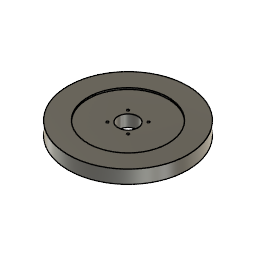
part - rotation base (Autodesk Fusion 360 design; units mm, degrees)
Autodesk Fusion 360 part; units mm, degrees
sketch "Sketch1" plane through (0, 0, 0) normal (0, 0, 1) x (1, 0, 0)
  circle A0 centre (0, 0) radius 90
  circle A1 centre (0, 0) radius 15
  line L0 (15.5, 15.5) -> (-15.5, 15.5)
  line L1 (-15.5, 15.5) -> (-15.5, -15.5)
  line L2 (-15.5, -15.5) -> (15.5, -15.5)
  line L3 (15.5, -15.5) -> (15.5, 15.5)
  line L4 (15.5, 15.5) -> (-15.5, -15.5) construction
  line L5 (-15.5, 15.5) -> (15.5, -15.5) construction
  circle A2 centre (-15.5, 15.5) radius 1.7
  circle A3 centre (15.5, 15.5) radius 1.7
  circle A4 centre (-15.5, -15.5) radius 1.7
  circle A5 centre (15.5, -15.5) radius 1.7
  dimension "d1" = 180
  dimension "d2" = 30
  dimension "d3" = 31
  dimension "d4" = 31
  dimension "d5" = 3.4
  dimension "d8" = 31
  dimension "d9" = -31
  constraint coincident A0.centre A1.centre
  constraint concentric A0 A1
  constraint horizontal L0
  constraint perpendicular L0 L1
  constraint parallel L0 L2
  constraint parallel L1 L3
  constraint coincident L4 A0.centre
  constraint coincident L5 A0.centre
  constraint coincident L0.end L1.start
  measures "d1" diameter of A0
  measures "d2" diameter of A1
  measures "d3" distance of L0.end L1.end
  measures "d4" distance of L0.start L0.end
  measures "d5" diameter of A2
extrude "Extrude1" add sketch "Sketch1" along normal blind 20 contours A0 | L0 L1 L2 L3 A2 A3 A4 A5
sketch "Sketch2" plane through (0, 0, 20) normal (0, 0, 1) x (-1, 0, 0)
  circle A0 centre (0, 0) radius 15
  circle A1 centre (15.5, -15.5) radius 1.7
  circle A2 centre (15.5, 15.5) radius 1.7
  circle A3 centre (-15.5, -15.5) radius 1.7
  circle A4 centre (-15.5, 15.5) radius 1.7
  circle A5 centre (0, 0) radius 90
  circle A6 centre (0, 0) radius 60.25
  dimension "d12" = 120.5
  constraint coincident A0.centre A5.centre
  measures "d12" diameter of A6
extrude "Extrude2" cut sketch "Sketch2" against normal blind 2.2 contours A6
hole "Hole1" at (15.5, -15.5, 0) direction (0, 0, 1) diameter 3.2 depth 17.8 tip angle 118 counterbore diameter 6.5 counterbore depth 5
hole "Hole2" at (15.5, 15.5, 0) direction (0, 0, 1) diameter 3.2 depth 17.8 tip angle 118 counterbore diameter 6.5 counterbore depth 5
hole "Hole3" at (-15.5, -15.5, 0) direction (0, 0, 1) diameter 3.2 depth 17.8 tip angle 118 counterbore diameter 6.5 counterbore depth 5
hole "Hole4" at (-15.5, 15.5, 0) direction (0, 0, 1) diameter 3.2 depth 17.8 tip angle 118 counterbore diameter 6.5 counterbore depth 5
